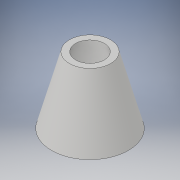
# Autodesk Inventor part: pressurechamber
Saved by Autodesk Inventor 2018 (Build 220112000, 112)
## iProperties
Created: 2018-04-21
Part Number: pressurechamber
Material: Generic
Document SubType Name: Modeling
Designer: atbin
Density: 0.231958 g/cm^3
Appearance: Default
Mass: 1.7787e+06 g
Surface Area: 577172 cm^2
Volume: 7.66819e+06 cm^3
Author: atbin
Autodesk Inventor part; units mm, degrees
ref_plane "YZ Plane" through (0, 0, 0) normal (1, 0, 0) x (0, 1, 0)
ref_plane "XZ Plane" through (0, 0, 0) normal (0, 1, 0) x (-1, 0, 0)
ref_plane "XY Plane" through (0, 0, 0) normal (0, 0, 1) x (1, 0, 0)
sketch "Sketch1" plane through (0, 0, 0) normal (0, 0, 1) x (1, 0, 0)
  line L0 (-1550, 0) -> (-1850, 0)
  line L1 (0, 3840) -> (0, -640) projected
  line L2 (0, 0) -> (3200, 0) construction
  line L3 (-1850, 0) -> (-992.5626, 3200)
  line L4 (-1850, 0) -> (1583.2735, 0) construction
  line L5 (-992.5626, 3200) -> (-692.5626, 3200)
  line L6 (-992.5626, 3200) -> (-692.5626, 3200) construction
  line L7 (-692.5626, 3200) -> (-1550, 0)
  dimension "d0" = 1850
  dimension "d5" = 75
  dimension "d6" = 300
  dimension "d7" = 0
  constraints: 14 end point, 4 horizontal, 1 collinear
  measures "d0" distance of L2.start L0.end
  measures "d5" angle of L4 L3
  measures "d6" distance of L3.end L5.end
  measures "d7" distance between parallel lines of L6 L5
revolve "Revolution1" add sketch "Sketch1" angle 360 about axis through (0, 0, 0) along (0, -1, 0)
body "Solid1"
